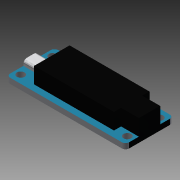
# Autodesk Inventor part: Board
Saved by Autodesk Inventor 2014 SP1 (Build 180222100, 222)
## iProperties
Created: 2014-04-30
Part Number: Board
Material: Generic
Document SubType Name: Modeling
Designer: david
Density: 1 g/cm^3
Appearance: Default
Author: david
Autodesk Inventor part; units mm, degrees
ref_plane "YZ Plane" through (0, 0, 0) normal (1, 0, 0) x (0, 1, 0)
ref_plane "XZ Plane" through (0, 0, 0) normal (0, 1, 0) x (-1, 0, 0)
ref_plane "XY Plane" through (0, 0, 0) normal (0, 0, 1) x (1, 0, 0)
sketch "Sketch1" plane through (0, 0, 0) normal (0, 1, 0) x (-1, 0, 0)
  line L0 (33.5, -13.5) -> (-33.5, -13.5)
  line L1 (-33.5, -13.5) -> (-33.5, 13.5)
  line L2 (-33.5, 13.5) -> (33.5, 13.5)
  line L3 (33.5, 13.5) -> (33.5, -13.5)
  line L4 (0, 0) -> (86.7229, 0) construction
  line L5 (0, 0) -> (0, 45.1017) construction
  dimension "d0" = 27
  dimension "d1" = 67
  constraints: 12 end point, 3 perpendicular, 2 parallel, 1 horizontal, 2 other
  measures "d0" distance of L0.end L1.end
  measures "d1" distance between parallel lines of L3 L1
extrude "Extrusion1" add sketch "Sketch1" along normal blind 3
sketch "Sketch2" plane through (0, 3, 0) normal (0, 1, 0) x (1, 0, 0)
  line L0 (33.5, 13.5) -> (-33.5, 13.5) projected
  line L1 (33.5, -13.5) -> (33.5, 13.5) projected
  line L2 (0, 0) -> (26.8835, 0) construction
  line L3 (0, 0) -> (0, 11.9949) construction
  circle A0 centre (30, 9) radius 2.15
  circle A1 centre (-30, 9) radius 2.15
  circle A2 centre (30, -9) radius 2.15
  circle A3 centre (-30, -9) radius 2.15
  dimension "d4" = 4.3
  dimension "d5" = 3.5
  dimension "d6" = 4.5
  constraints: 4 centre point, 4 end point, 3 symmetric about line, 2 perpendicular, 3 other
  measures "d4" diameter of A0
  measures "d5" distance from line of L1 A0.centre
  measures "d6" distance from line of A0.centre L0
extrude "Extrusion2" cut sketch "Sketch2" against normal through all
fillet "Fillet1" radius 2 4 edges at (-33.5, 1.5, 13.5) (-33.5, 1.5, -13.5) (33.5, 1.5, -13.5) (33.5, 1.5, 13.5)
sketch "Sketch3" plane through (0, 3, 0) normal (0, 1, 0) x (1, 0, 0)
  line L0 (33.5, -11.5) -> (33.5, 11.5) projected
  line L1 (23.5, 6) -> (33.5, 6)
  line L2 (33.5, 6) -> (33.5, -6)
  line L3 (33.5, -6) -> (23.5, -6)
  line L4 (23.5, -6) -> (23.5, 6)
  line L5 (0, 0) -> (50.7888, 0) construction
  line L6 (23.5, 10) -> (-21.5, 10)
  line L7 (-21.5, 10) -> (-21.5, -10)
  line L8 (-21.5, -10) -> (23.5, -10)
  line L9 (23.5, -10) -> (23.5, 10)
  dimension "d10" = 10
  dimension "d11" = 12
  dimension "d12" = 20
  dimension "d13" = 45
  constraints: 18 end point, 4 parallel, 3 perpendicular, 2 collinear, 2 horizontal, 2 other
  measures "d10" distance between parallel lines of L2 L4
  measures "d11" distance between parallel lines of L3 L1
  measures "d12" distance between parallel lines of L8 L6
  measures "d13" distance between parallel lines of L9 L7
extrude "Extrusion3" add sketch "Sketch3" along normal blind 9
sketch "Sketch4" plane through (0, 3, 0) normal (0, 1, 0) x (1, 0, 0)
  line L0 (-33.5, 11.5) -> (-33.5, -11.5) projected
  line L1 (-33.5, 4) -> (-27.5, 4)
  line L2 (-27.5, 4) -> (-27.5, -4)
  line L3 (-27.5, -4) -> (-33.5, -4)
  line L4 (-33.5, -4) -> (-33.5, 4)
  line L5 (0, 0) -> (-50.5157, 0) construction
  dimension "d16" = 6
  dimension "d17" = 8
  constraints: 10 end point, 2 parallel, 2 perpendicular, 1 horizontal, 1 point on line, 1 other
  measures "d16" distance between parallel lines of L4 L2
  measures "d17" distance between parallel lines of L3 L1
extrude "Extrusion4" add sketch "Sketch4" along normal blind 3
fillet "Fillet2" radius 2 2 edges at (-30.5, 6, 4) (-30.5, 6, -4)
body "Solid1"
